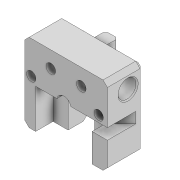
# Autodesk Inventor part: Print_Parts_S
Saved by Autodesk Inventor 2020.1 (Build 241239000, 239)
## iProperties
Created: 2020-11-09
Part Number: Print_Parts_S
Material: 一般
Document SubType Name: Modeling
Designer: kenta iguchi
Density: 1 g/cm^3
Appearance: 既定
Author: kenta iguchi
Autodesk Inventor part; units mm, degrees
ref_plane "YZ Plane" through (0, 0, 0) normal (1, 0, 0) x (0, 1, 0)
ref_plane "XZ Plane" through (0, 0, 0) normal (0, 1, 0) x (-1, 0, 0)
ref_plane "XY Plane" through (0, 0, 0) normal (0, 0, 1) x (1, 0, 0)
sketch "スケッチ1" plane through (0, 0, 0) normal (0, 0, 1) x (1, 0, 0)
  line L0 (0, 0) -> (30, 0)
  line L1 (30, 0) -> (30, 30)
  line L2 (30, 30) -> (0, 30)
  line L3 (0, 30) -> (0, 0)
  line L4 (3.9, 0) -> (16.1, 0)
  line L5 (16.1, 0) -> (16.1, 10.3588)
  line L6 (16.1, 10.3588) -> (3.9, 10.3588)
  line L7 (3.9, 10.3588) -> (3.9, 0)
  point P0 (10, 10.3588)
  point P1 (16.1, 0)
  dimension "d0" = 30
  dimension "d1" = 12.2
  dimension "d2" = 10
  dimension "d3" = 30
  constraints: 16 end point, 4 parallel, 2 horizontal, 2 perpendicular, 1 midpoint, 1 point on line
  measures "d0" distance of L1.end L2.end
  measures "d1" distance of L5.end L6.end
  measures "d2" distance from line of point (10, 10.359) L3
  measures "d3" distance of L0.end L1.end
extrude "押し出し1" add sketch "スケッチ1" along normal blind 20 contours L3 L2 L1 L0 L5 L6 L7
sketch "スケッチ2" plane through (0, 0, 20) normal (0, 0, 1) x (1, 0, 0)
  line L0 (0, 30) -> (0, 0) projected
  line L1 (0, 0) -> (-8, 0)
  line L2 (-8, 0) -> (-8, 30)
  line L3 (-8, 30) -> (0, 30)
  line L4 (0, 30) -> (0, 0)
  dimension "d6" = 8
  constraints: 8 end point, 2 parallel, 1 horizontal, 1 horizontal alignment, 1 perpendicular
  measures "d6" distance of L2.end L3.end
extrude "押し出し2" add sketch "スケッチ2" against normal blind 40
sketch "スケッチ4" plane through (0, 0, 20) normal (0, 0, 1) x (1, 0, 0)
  line L0 (16.1, 0) -> (30, 0) projected
  line L1 (-8, 0) -> (3.9, 0) projected
  line L2 (3.9, 0) -> (3.9, 10.3588) projected
  line L3 (3.9, 10.3588) -> (16.1, 10.3588) projected
  line L4 (16.1, 10.3588) -> (16.1, 0) projected
  line L5 (-2.1, -6.2) -> (22.1, -6.2)
  line L6 (22.1, -6.2) -> (22.1, 12)
  line L7 (22.1, 12) -> (-2.1, 12)
  line L8 (-2.1, 12) -> (-2.1, -6.2)
  point P0 (0, 0)
  point P1 (10, 10.3588)
  point P2 (10, -6.2)
  point P3 (10, 10.3588)
  point P4 (22.1, 0)
  point P5 (-2.1, 0)
  dimension "d14" = 24.2
  dimension "d15" = 18.2
  dimension "d16" = 12
  constraints: 8 end point, 3 midpoint, 2 parallel, 1 horizontal, 1 perpendicular, 1 vertical alignment
  measures "d14" distance of L7.end L6.end
  measures "d15" distance of L6.end L5.end
  measures "d16" distance between parallel lines of L7 L1
extrude "押し出し4" cut sketch "スケッチ4" against normal blind 11 contours L4 L3 L2 L1 L8 L7 L6 L0
sketch "スケッチ5" plane through (0, 0, 9) normal (0, 0, 1) x (1, 0, 0)
  line L0 (-2.1, 0) -> (-2.1, 12) projected
  line L1 (22.1, 12) -> (22.1, 0) projected
  line L2 (-2.1, 12) -> (22.1, 12) projected
  point P0 (0, 0)
  point P1 (0.5, 9.1)
  point P2 (19.5, 9.1)
  dimension "d19" = 2.6
  dimension "d20" = 2.6
  dimension "d21" = 2.9
  constraints: 1 horizontal alignment
  measures "d19" distance from line of point (0.5, 9.1) L0
  measures "d20" distance from line of L1 point (19.5, 9.1)
  measures "d21" distance from line of L2 point (19.5, 9.1)
hole "穴1" at (0.5, 9.1, 9) at (19.5, 9.1, 9) direction (0, 0, -1) diameter 4.4 depth 6
sketch "スケッチ6" plane through (0, 0, 20) normal (0, 0, 1) x (1, 0, 0)
  line L0 (-2.1, 0) -> (-2.1, 12) projected
  line L1 (-2.1, 12) -> (22.1, 12) projected
  line L2 (22.1, 12) -> (22.1, 0) projected
  line L3 (22.1, 0) -> (30, 0) projected
  line L4 (30, 0) -> (30, 30) projected
  line L5 (30, 30) -> (-8, 30) projected
  line L6 (-8, 30) -> (-8, 0) projected
  line L7 (-8, 0) -> (-2.1, 0) projected
  point P0 (0, 0)
extrude "押し出し5" cut sketch "スケッチ6" against normal blind 5
sketch "スケッチ7" plane through (30, 0, 0) normal (1, 0, 0) x (0, 0, -1)
  line L0 (-15, 30) -> (-15, 0) projected
  line L1 (0, 30) -> (-15, 30) projected
  circle A0 centre (-7.5, 22.5) radius 4.15
  dimension "d31" = 8.3
  dimension "d32" = 7.5
  dimension "d33" = 7.5
  constraints: 1 centre point
  measures "d31" diameter of A0
  measures "d32" distance from line of L0 A0.centre
  measures "d33" distance from line of L1 A0.centre
extrude "押し出し6" cut sketch "スケッチ7" against normal through all
sketch "スケッチ8" plane through (0, 0, 0) normal (0, -1, 0) x (1, 0, 0)
  line L0 (-2.1, 15) -> (-8, 15) projected
  line L1 (-8, 15) -> (-8, -20) projected
  line L2 (0, -20) -> (-8, -20) projected
  line L3 (0, 0) -> (0, -20) projected
  line L4 (0, 0) -> (3.9, 0) projected
  line L5 (3.9, 0) -> (3.9, 9) projected
  line L6 (3.9, 9) -> (-2.1, 9) projected
  line L7 (-2.1, 9) -> (-2.1, 15) projected
  line L8 (30, 15) -> (22.1, 15) projected
  line L9 (22.1, 15) -> (22.1, 9) projected
  line L10 (22.1, 9) -> (16.1, 9) projected
  line L11 (16.1, 0) -> (16.1, 9) projected
  line L12 (16.1, 0) -> (30, 0) projected
  line L13 (30, 0) -> (30, 15) projected
extrude "押し出し7" add sketch "スケッチ8" along normal blind 6
sketch "スケッチ11" plane through (0, 0, 15) normal (0, 0, 1) x (1, 0, 0)
  line L0 (22.1, -6) -> (22.1, 12) projected
  line L1 (30, 30) -> (30, -6) projected
  line L2 (22.1, 12) -> (30, 12)
  line L3 (30, 12) -> (30, 7)
  line L4 (30, 7) -> (22.1, 7)
  line L5 (22.1, 7) -> (22.1, 12)
  point P0 (0, 0)
  dimension "d45" = 5
  constraints: 8 end point, 2 parallel, 1 horizontal, 1 perpendicular, 1 point on line
  measures "d45" distance between parallel lines of L2 L4
extrude "押し出し10" cut sketch "スケッチ11" against normal up to surface (6 mm away)
sketch "スケッチ12" plane through (0, 0, 15) normal (0, 0, 1) x (1, 0, 0)
  line L0 (30, 12) -> (-2.1, 12) projected
  line L1 (30, 30) -> (30, 12) projected
  line L2 (-8, 30) -> (30, 30) projected
  line L3 (-8, -6) -> (-8, 30) projected
  line L4 (-2.1, -6) -> (-8, -6) projected
  line L5 (-2.1, 12) -> (-2.1, -6) projected
  line L6 (30, 7) -> (22.1, 7) projected
  line L7 (22.1, -6) -> (22.1, 7) projected
  line L8 (30, -6) -> (22.1, -6) projected
  line L9 (30, 7) -> (30, -6) projected
  point P0 (0, 0)
extrude "押し出し11" add sketch "スケッチ12" along normal blind 2
sketch "スケッチ13" plane through (0, 0, 17) normal (0, 0, 1) x (1, 0, 0)
  line L0 (30, 26.65) -> (30, 18.35) projected
  line L1 (-8, 18.35) -> (-8, 26.65) projected
  line L2 (-8, 22.5) -> (30, 22.5)
  point P0 (0, 0)
  point P1 (4, 22.5)
  point P2 (18, 22.5)
  dimension "d51" = 14
  dimension "d78" = 12
  constraints: 2 end point, 2 midpoint, 2 point on line
  measures "d51" distance of point (18, 22.5) point (4, 22.5)
  measures "d78" horizontal distance of point (4, 22.5) L1.end
hole "穴2" at (4, 22.5, 17) at (18, 22.5, 17) direction (0, 0, -1) diameter 4.4 depth 6
sketch "スケッチ14" plane through (-8, -6, -20) normal (-1, 0, 0) x (0, 0, 1)
  line L0 (37, 36) -> (0, 36) projected
  line L1 (0, 36) -> (0, 0) projected
  line L2 (0, 0) -> (37, 0) projected
  line L3 (20, 36) -> (20, 0) projected
  line L4 (0, 0) -> (20, 0) projected
  line L5 (0, 36) -> (0, 0) projected
  line L6 (20, 36) -> (0, 36) projected
  point P0 (20, 6)
  point P1 (10, 28)
  point P2 (10, 8)
  dimension "d59" = 10
  dimension "d60" = 8
  dimension "d61" = 8
  constraints: 1 vertical alignment
  measures "d59" distance from line of point (10, 28) L1
  measures "d60" distance from line of point (10, 28) L0
  measures "d61" distance from line of L2 point (10, 8)
hole "穴3" at (-8, 22, -10) at (-8, 2, -10) direction (1, 0, 0) diameter 4.3 depth 6 counterbore diameter 8 counterbore depth 4
chamfer "面取り1" distance 0.5 angle 45 4 edges at (-8, 22.5, 11.65) (-8, 22, -14) (-8, 2, -14) (30, 22.5, 11.65)
chamfer "面取り3" distance 5 angle 45 1 edges at (30, 9.5, 9)
sketch "スケッチ15" plane through (0, 0, 17) normal (0, 0, 1) x (1, 0, 0)
  line L0 (-8, 30) -> (-8, -6) projected
  line L1 (22.1, 7) -> (22.1, -6) projected
  line L2 (22.1, -6) -> (30, -6) projected
  line L3 (30, -6) -> (30, 7) projected
  line L4 (30, 7) -> (22.1, 7) projected
  point P0 (0, 0)
  point P1 (-5, 15)
  point P2 (26, -1)
  point P3 (-5, -1)
  point P4 (26, 15)
  dimension "d79" = 5
  dimension "d80" = 4
  dimension "d81" = 3
  dimension "d82" = 16
  constraints: 2 horizontal alignment, 2 vertical alignment
  measures "d79" distance from line of point (26, -1) L2
  measures "d80" distance from line of point (26, -1) L3
  measures "d81" distance from line of point (-5, -1) L0
  measures "d82" distance of point (-5, 15) point (-5, -1)
hole "穴4" at (-5, 15, 17) at (26, 15, 17) direction (0, 0, -1) diameter 4.3 depth 6
chamfer "面取り4" distance 2 angle 45 5 edges at (-8, 30, -1.5) (-8, 12, -20) (-8, -6, -1.5) (30, 30, 8.5) (30, -6, 8.5)
sketch "スケッチ17" plane through (0, 30, 0) normal (1, 0, 0) x (0, 0, -1)
  line L0 (0, 0) -> (0, -36) projected
  line L1 (20, -36) -> (0, -36) projected
  line L2 (20, 0) -> (20, -36) projected
  line L3 (0, 0) -> (20, 0) projected
  line L4 (0, -36) -> (20, -36)
  line L5 (20, -36) -> (20, 0)
  line L6 (20, 0) -> (0, 0)
  line L7 (0, 0) -> (0, -36)
  point P0 (0, -30)
  dimension "d93" = 20
  constraints: 8 end point, 2 parallel, 1 horizontal, 1 perpendicular
  measures "d93" distance of L6.end L2.start
extrude "押し出し12" cut sketch "スケッチ17" against normal blind 10
sketch "スケッチ18" plane through (0, 0, 9) normal (0, 0, 1) x (1, 0, 0)
  line L0 (3.9, 10.3588) -> (3.9, -6) projected
  line L1 (16.1, 10.3588) -> (3.9, 10.3588) projected
  line L2 (16.1, 10.3588) -> (16.1, -6) projected
  line L3 (3.9, 10.3588) -> (3.9, -6) projected
  line L4 (3.9, 10.3588) -> (16.1, 10.3588)
  line L5 (16.1, 10.3588) -> (16.1, 6.3588)
  line L6 (16.1, 6.3588) -> (3.9, 6.3588)
  line L7 (3.9, 6.3588) -> (3.9, 10.3588)
  point P0 (0, 0)
  point P1 (3.9, 6.3588)
  dimension "d96" = 4
  constraints: 8 end point, 2 parallel, 1 horizontal, 1 perpendicular, 1 point on line
  measures "d96" distance between parallel lines of L1 L6
extrude "押し出し13" add sketch "スケッチ18" against normal up to surface (9 mm away)
sketch "スケッチ19" plane through (0, 0, 17) normal (0, 0, 1) x (1, 0, 0)
  line L0 (3.9, 6.3588) -> (16.1, 6.3588) projected
  point P0 (0, 0)
  point P1 (10, 6.3588)
  point P2 (10, 11.3588)
  dimension "d99" = 5
  constraints: 1 midpoint
  measures "d99" distance from line of point (10, 11.359) L0
hole "穴5" at (10, 11.3588, 17) direction (0, 0, -1) diameter 3.3 end through all counterbore diameter 6.5 counterbore depth 12
chamfer "面取り5" distance 2 angle 45 9 edges at (11, 30, 0) (-7, 29, 0) (-8, 12, 0) (-7, -5, 0) (-1.05, -6, 0) (22.05, -6, 0) (29, -5, 0) (30, 12, 0) (29, 29, 0)
sketch "スケッチ20" plane through (0, 0, 0) normal (0, 0, -1) x (-1, 0, 0)
  line L0 (-27.1716, 28) -> (5.1716, 28) projected
  circle A0 centre (-10, 11.3588) radius 1.65 projected
  line L1 (-12.9, 28) -> (-7.1, 28)
  line L2 (-7.1, 28) -> (-7.1, 19.3588)
  line L3 (-7.1, 19.3588) -> (-12.9, 19.3588)
  line L4 (-12.9, 19.3588) -> (-12.9, 28)
  point P0 (0, 0)
  dimension "d112" = 2.9
  dimension "d114" = 8
  constraints: 8 end point, 2 parallel, 1 horizontal, 1 perpendicular, 1 point on line
  measures "d112" distance from line of L2 A0.centre
  measures "d114" distance from line of L3 A0.centre
extrude "押し出し14" add sketch "スケッチ20" along normal blind 5 contours L0 L2 L3 L4
chamfer "面取り6" distance 1 angle 45 5 edges at (7.1, 23.6794, -5) (12.9, 23.6794, -5) (7.1, 19.3588, -2.5) (10, 19.3588, -5) (12.9, 19.3588, -2.5)
sketch "スケッチ21" plane through (0, -6, 0) normal (0, -1, 0) x (1, 0, 0)
  line L0 (3.9, 9) -> (-2.1, 9) projected
  line L1 (-3, 9) -> (23, 9)
  line L2 (23, 9) -> (23, 11)
  line L3 (23, 11) -> (-3, 11)
  line L4 (-3, 11) -> (-3, 9)
  line L5 (3.9, 9) -> (16.1, 9) projected
  point P0 (0, 0)
  point P1 (10, 9)
  dimension "d120" = 26
  dimension "d121" = 13
  dimension "d122" = 2
  constraints: 8 end point, 2 parallel, 1 horizontal, 1 horizontal alignment, 1 midpoint, 1 perpendicular
  measures "d120" distance of L2.end L3.end
  measures "d121" distance from line of point (10, 9) L4
  measures "d122" distance of L3.end L1.start
extrude "押し出し15" cut sketch "スケッチ21" against normal up to surface (18 mm away)
sketch "スケッチ22" plane through (0, 0, 17) normal (0, 0, 1) x (1, 0, 0)
  arc A0 (13.1861, 12) -> (6.8139, 12) centre (10, 11.3588) ccw projected
  line L0 (13.1861, 12) -> (30, 12) projected
  line L1 (-6, -6) -> (-2.1, -6) projected
  line L2 (-2.1, 12) -> (6.8139, 12) projected
  line L3 (25, 12) -> (13.1861, 12) projected
  line L4 (-3, -6) -> (23, -6)
  line L5 (23, -6) -> (23, 12)
  line L6 (23, 12) -> (-3, 12)
  line L7 (-3, 12) -> (-3, -6)
  point P0 (0, 0)
  point P1 (6.8139, 12)
  dimension "d128" = 26
  dimension "d129" = 13
  constraints: 8 end point, 2 parallel, 2 point on line, 1 horizontal, 1 perpendicular
  measures "d128" distance of L5.end L6.end
  measures "d129" distance from line of L5 A0.centre
extrude "押し出し16" cut sketch "スケッチ22" against normal up to surface (8 mm away) contours L0 L5 L4 L1 L7 L6 L2
equation "\"d112\" = 0.5 * d111"
equation "\"d111\" = 5.8"
